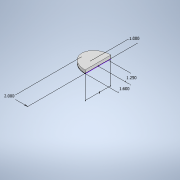
# Autodesk Inventor part: pryBarHolder
Saved by Autodesk Inventor 2021 (Build 250183000, 183)
## iProperties
Created: 2020-06-10
Part Number: pryBarHolder
Material: Generic
Document SubType Name: Modeling
Designer: robst
Density: 1 g/cm^3
Appearance: Default
Author: robst
Autodesk Inventor part; units mm, degrees
ref_plane "YZ Plane" through (0, 0, 0) normal (1, 0, 0) x (0, 1, 0)
ref_plane "XZ Plane" through (0, 0, 0) normal (0, 1, 0) x (-1, 0, 0)
ref_plane "XY Plane" through (0, 0, 0) normal (0, 0, 1) x (1, 0, 0)
sketch "Sketch1" plane through (0, 0, 0) normal (0, 1, 0) x (-1, 0, 0)
  ellipse E0 centre (0, 0) end of major axis (0, -40.64) minor radius 50.8 (0, -40.64) -> (0, 40.64) ccw
  line L0 (0, 40.64) -> (0, -40.64)
  ellipse E1 centre (0, 0) end of major axis (0, -31.75) minor radius 25.4 (0, -31.75) -> (0, 31.75) ccw
  line L1 (0, 40.64) -> (0, -40.64)
  point P0 (0, -31.75)
  point P1 (0, 31.75)
  dimension "d0" = 50.8
  dimension "d1" = 40.64
  dimension "d2" = 25.4
  dimension "d3" = 31.75
  constraints: 4 end point, 2 coincident, 2 point on line, 2 vertical, 8 other
extrude "Extrusion1" add sketch "Sketch1" along normal blind 9.525
extrude "Extrusion2" add sketch "Sketch1" against normal blind 9.525 contours L0 E1
sketch "Sketch3" plane through (0, -9.525, 0) normal (0, -1, 0) x (1, 0, 0)
  line L0 (0, -31.75) -> (0, 31.75) projected
  ellipse E0 centre (0, 0) end of major axis (0, -31.75) minor radius 25.4 (0, 31.75) -> (0, -31.75) ccw projected
  line L1 (0, 40.64) -> (0, -40.64) projected
  ellipse E1 centre (0, 0) end of major axis (0, -31.75) minor radius 25.4 (0, 31.75) -> (0, -31.75) ccw projected
  line L2 (-9.525, 29.433) -> (-9.525, -29.433)
  ellipse E2 centre (0, 0) end of major axis (0, -31.75) minor radius 25.4 (0, 31.75) -> (-9.525, 29.433) ccw
  ellipse E3 centre (0, 0) end of major axis (0, -31.75) minor radius 25.4 (-9.525, -29.433) -> (0, -31.75) ccw
  point P0 (-9.525, -29.433)
  dimension "d8" = 9.525
  constraints: 4 vertical, 2 end point, 2 point on line, 1 coincident, 12 other
  measures "d8" distance between parallel lines of L2 L0
extrude "Extrusion3" cut sketch "Sketch3" against normal blind 9.525 contours E0 L2 L0
body "Solid1"
